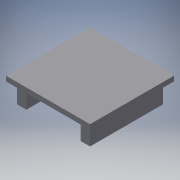
# Autodesk Inventor part: hull_cover_cover
Saved by Autodesk Inventor 2018 (Build 220112000, 112)
## iProperties
Created: 2018-01-11
Part Number: hull_cover_cover
Material: Generic
Document SubType Name: Modeling
Designer: erwin
Density: 1 g/cm^3
Appearance: Default
Author: erwin
Autodesk Inventor part; units mm, degrees
ref_plane "YZ Plane" through (0, 0, 0) normal (1, 0, 0) x (0, 1, 0)
ref_plane "XZ Plane" through (0, 0, 0) normal (0, 1, 0) x (-1, 0, 0)
ref_plane "XY Plane" through (0, 0, 0) normal (0, 0, 1) x (1, 0, 0)
sketch "Sketch1" plane through (0, 0, 0) normal (0, 0, 1) x (1, 0, 0)
  line L0 (7.5, 7.5) -> (-7.5, 7.5) projected
  line L1 (7.5, 7.5) -> (-7.5, 7.5) projected
  line L2 (-7.5, 7.5) -> (-7.5, -7.5) projected
  line L3 (-7.5, -7.5) -> (7.5, -7.5) projected
  line L4 (7.5, -7.5) -> (7.5, 7.5) projected
  line L5 (-8.5, 8.5) -> (8.5, 8.5) projected
  line L6 (8.5, 8.5) -> (8.5, -8.5) projected
  line L7 (8.5, -8.5) -> (-8.5, -8.5) projected
  line L8 (-8.5, -8.5) -> (-8.5, 8.5) projected
  point P0 (0, 0)
extrude "Extrusion1" add sketch "Sketch1" along normal blind 1 contours L4 L3 L2 L0 | L5 L6 L7 L8
sketch "Sketch2" plane through (0, 0, 0) normal (0, 0, -1) x (-1, 0, 0)
  line L0 (-7.5, 7.5) -> (7.5, 7.5) projected
  line L1 (7.5, 7.5) -> (7.5, -7.5) projected
  line L2 (7.5, -7.5) -> (-7.5, -7.5) projected
  line L3 (-7.5, -7.5) -> (-7.5, 7.5) projected
  line L4 (8.5, 8.5) -> (-8.5, 8.5) projected
  line L5 (-8.5, 8.5) -> (-8.5, -8.5) projected
  line L6 (-8.5, -8.5) -> (8.5, -8.5) projected
  line L7 (8.5, -8.5) -> (8.5, 8.5) projected
  line L8 (-7.5, -7.5) -> (-5.5, -7.5)
  line L9 (-5.5, -7.5) -> (-5.5, 7.5)
  line L10 (-5.5, 7.5) -> (-7.5, 7.5)
  line L11 (-7.5, 7.5) -> (-7.5, -7.5)
  line L12 (7.5, 7.5) -> (5.5, 7.5)
  line L13 (5.5, 7.5) -> (5.5, -7.5)
  line L14 (5.5, -7.5) -> (7.5, -7.5)
  line L15 (7.5, -7.5) -> (7.5, 7.5)
  point P0 (0, 0)
  dimension "d2" = 2
  dimension "d3" = 2
  constraints: 16 end point, 4 parallel, 2 horizontal, 2 perpendicular, 2 point on line
  measures "d2" distance of L10.end L9.end
  measures "d3" distance of L14.end L13.end
extrude "Extrusion2" add sketch "Sketch2" along normal blind 4 contours L0 L9 L2 L3 | L0 L1 L2 L13
thicken "Thicken1" operation add thickness 0.1 both sides no extend neighbours yes toward (0, -1, 0) faces at (6.1667, 7.5, -1.3333) (7.5, 2.5, -1.3333) (6.8333, -7.5, -1.3333)
thicken "Thicken2" operation add thickness 0.1 both sides no extend neighbours yes toward (0, 1, 0) faces at (-6.1667, -7.5, -1.3333) (-7.5, -2.5, -1.3333) (-6.8333, 7.5, -1.3333)
body "Solid1"
